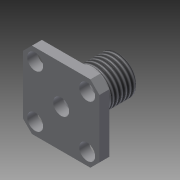
# Autodesk Inventor part: SMA_connector
Saved by Autodesk Inventor 2015 (Build 190159000, 159)
## iProperties
Created: 2014-11-11
Part Number: SMA_connector
Material: Generic
Document SubType Name: Modeling
Designer: Alexander
Density: 1 g/cm^3
Appearance: Vorgabe
Author: Alexander
Autodesk Inventor part; units mm, degrees
ref_plane "YZ Plane" through (0, 0, 0) normal (1, 0, 0) x (0, 1, 0)
ref_plane "XZ Plane" through (0, 0, 0) normal (0, 1, 0) x (-1, 0, 0)
ref_plane "XY Plane" through (0, 0, 0) normal (0, 0, 1) x (1, 0, 0)
sketch "Sketch1" plane through (0, 0, 0) normal (0, 1, 0) x (-1, 0, 0)
  line L0 (4.85, 6.35) -> (-4.85, 6.35)
  line L1 (-6.35, 4.85) -> (-6.35, -4.85)
  line L2 (-4.85, -6.35) -> (4.85, -6.35)
  line L3 (6.35, -4.85) -> (6.35, 4.85)
  line L4 (6.35, 6.35) -> (-6.35, -6.35) construction
  line L5 (-6.35, 6.35) -> (6.35, -6.35) construction
  line L6 (6.35, -4.85) -> (4.85, -6.35)
  line L7 (-4.85, -6.35) -> (-6.35, -4.85)
  line L8 (-4.85, 6.35) -> (-6.35, 4.85)
  line L9 (6.35, 4.85) -> (4.85, 6.35)
  line L10 (4.32, 4.32) -> (-4.32, 4.32) construction
  line L11 (-4.32, 4.32) -> (-4.32, -4.32) construction
  line L12 (-4.32, -4.32) -> (4.32, -4.32) construction
  line L13 (4.32, -4.32) -> (4.32, 4.32) construction
  line L14 (4.32, 4.32) -> (-4.32, -4.32) construction
  line L15 (-4.32, 4.32) -> (4.32, -4.32) construction
  circle A0 centre (0, 0) radius 1.3272
  dimension "d0" = 12.7
  dimension "d1" = 12.7
  dimension "d5" = 9.7
  dimension "d6" = 1.5
  dimension "d7" = 8.64
  dimension "d8" = 8.64
  dimension "d9" = 2.6543
  constraints: 32 end point, 8 point on line, 6 coincident, 4 midpoint, 4 parallel, 2 horizontal, 2 perpendicular, 1 centre point
  measures "d0" distance of L5.end L4.end
  measures "d1" distance of L4.end L5.start
  measures "d5" distance of L3.end L3.start
  measures "d6" horizontal distance of L3.end L0.start
  measures "d7" distance of L12.end L11.end
  measures "d8" distance of L11.end L10.end
  measures "d9" diameter of A0
extrude "Extrusion1" add sketch "Sketch1" along normal blind 1.65
sketch "Sketch2" plane through (0, 1.65, 0) normal (0, 1, 0) x (1, 0, 0)
  circle A0 centre (0, 0) radius 1.3272 projected
  line L0 (-4.32, -4.32) -> (4.32, -4.32) construction
  line L1 (4.32, -4.32) -> (4.32, 4.32) construction
  line L2 (4.32, 4.32) -> (-4.32, 4.32) construction
  line L3 (-4.32, 4.32) -> (-4.32, -4.32) construction
  line L4 (-4.32, -4.32) -> (4.32, 4.32) construction
  line L5 (4.32, -4.32) -> (-4.32, 4.32) construction
  dimension "d12" = 8.64
  dimension "d13" = 8.64
  constraints: 12 end point, 4 coincident, 2 midpoint, 2 parallel, 1 horizontal, 1 perpendicular
  measures "d12" distance of L2.end L1.end
  measures "d13" distance of L1.end L0.end
hole "Hole1" at (-4.32, 1.65, -4.32) at (4.32, 1.65, -4.32) at (4.32, 1.65, 4.32) at (-4.32, 1.65, 4.32) direction (0, -1, 0) diameter 2.64 depth 1.65 tip angle 118
sketch "Sketch3" plane through (0, 1.65, 0) normal (0, 1, 0) x (1, 0, 0)
  circle A0 centre (0, 0) radius 1.3272 projected
  circle A1 centre (0, 0) radius 3.145
  dimension "d21" = 6.29
  constraints: 1 centre point, 1 coincident
  measures "d21" diameter of A1
extrude "Extrusion2" add sketch "Sketch3" along normal blind 7.93 contours A0 | A1
thread "Thread1" size "1/4-36 UNS" class "2A" standard "ANSI Unified Screw Threads" length 4.38
chamfer "Chamfer1" distance 0.3 angle 45 1 edges at (-3.145, 9.58, 0)
sketch "Sketch4" plane through (0, 9.58, 0) normal (0, 1, 0) x (1, 0, 0)
  circle A0 centre (0, 0) radius 2.845 projected
  circle A1 centre (0, 0) radius 2.75
  dimension "d30" = 5.5
  constraints: 1 centre point, 1 coincident
  measures "d30" diameter of A1
extrude "Extrusion3" cut sketch "Sketch4" against normal blind 3 contours A1
sketch "Sketch5" plane through (0, 1.65, 0) normal (0, -1, 0) x (1, 0, 0)
  circle A0 centre (0, 0) radius 1.3272 projected
  circle A1 centre (0, 0) radius 0.254
  dimension "d33" = 0.508
  constraints: 1 centre point, 1 coincident
  measures "d33" diameter of A1
extrude "Extrusion4" cut sketch "Sketch5" against normal blind 6 contours A1
sketch "Sketch6" plane through (0, 6.58, 0) normal (0, 1, 0) x (1, 0, 0)
  circle A0 centre (0, 0) radius 0.254 projected
  circle A1 centre (0, 0) radius 2.75 projected
  circle A2 centre (0, 0) radius 0.5
  dimension "d36" = 1
  constraints: 1 centre point, 1 coincident
  measures "d36" diameter of A2
extrude "Extrusion5" cut sketch "Sketch6" against normal blind 2 contours A2
body "Solid1"
